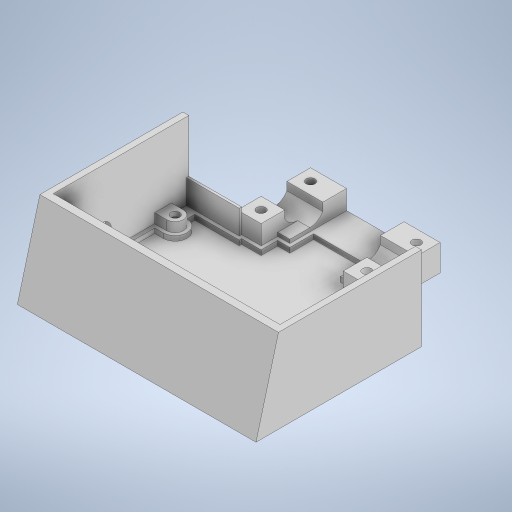
# Autodesk Inventor part: tělo estonsko
Saved by Autodesk Inventor 2024 (Build 280153000, 153)
## iProperties
Created: 2023-09-06
Part Number: tělo estonsko
Material: Všeobecné
Document SubType Name: Modeling
Designer: Simak
Density: 1 g/cm^3
Appearance: Výchozí
Author: Simak
Autodesk Inventor part; units mm, degrees
ref_plane "YZ Plane" through (0, 0, 0) normal (1, 0, 0) x (0, 1, 0)
ref_plane "XZ Plane" through (0, 0, 0) normal (0, 1, 0) x (-1, 0, 0)
ref_plane "XY Plane" through (0, 0, 0) normal (0, 0, 1) x (1, 0, 0)
sketch "Náčrt1" plane through (0, 0, 0) normal (0, 1, 0) x (-1, 0, 0)
  line L0 (49.75, -19.25) -> (49.75, 49.75)
  line L1 (49.75, 49.75) -> (-49.75, 49.75)
  line L2 (-49.75, 49.75) -> (-49.75, -19.25)
  line L3 (-49.75, -19.25) -> (-27, -19.25)
  line L4 (-27, -19.25) -> (-27, -49.75)
  line L5 (-27, -49.75) -> (27, -49.75)
  line L6 (27, -49.75) -> (27, -19.25)
  line L7 (27, -19.25) -> (49.75, -19.25)
  point P0 (0, 0)
  dimension "d0" = 30.5
  dimension "d1" = 99.5
  dimension "d2" = 22.75
  dimension "d3" = 99.5
  dimension "d4" = 54
  dimension "d5" = 49.75
  dimension "d6" = 49.75
  constraints: 16 end point, 6 perpendicular, 2 vertical, 1 parallel
  measures "d0" distance of L3.end L4.end
  measures "d1" distance of L0.end L1.end
  measures "d2" distance of L2.end L3.end
  measures "d3" distance between parallel lines of L1 L5
  measures "d4" distance of L4.end L5.end
  measures "d5" horizontal distance of L1.end point (0, 0)
  measures "d6" distance from line of point (0, 0) L1
extrude "Vysunutí1" add sketch "Náčrt1" along normal blind 3
sketch "Náčrt2" plane through (27, 0, -19.25) normal (1, 0, 0) x (0, 0, -1)
  line L0 (30.5, 3) -> (0, 3)
  line L1 (0, 3) -> (0, 11)
  line L2 (0, 11) -> (9.875, 11)
  line L3 (9.875, 11) -> (9.875, 7.646)
  arc A0 (9.875, 7.646) -> (20.625, 7.646) centre (15.25, 10.582835) ccw
  line L4 (20.625, 7.646) -> (20.625, 11)
  line L5 (20.625, 11) -> (30.5, 11)
  line L6 (30.5, 11) -> (30.5, 3)
  line L7 (0, 0) -> (30.5, 0)
  point P0 (-19.25, 0)
  dimension "d9" = 6.125
  dimension "d10" = 11
  dimension "d11" = 9.875
  dimension "d12" = 3.354
  constraints: 12 end point, 3 perpendicular, 2 equal length, 2 point on circle, 2 point on line, 1 centre point, 1 parallel, 1 vertical
  measures "d9" radius of A0
  measures "d10" distance between parallel lines of L5 L7
  measures "d11" distance of L4.end L5.end
  measures "d12" distance of L4.start L4.end
extrude "Vysunutí2" add sketch "Náčrt2" against normal up to surface (54 mm away)
sketch "Náčrt3" plane through (27, 3, -19.25) normal (0, 0, 1) x (1, 0, 0)
  line L0 (0, 8) -> (-54, 8) projected
  line L1 (-39, 8) -> (-39, 0)
  line L2 (-15, 8) -> (-15, 0)
  line L3 (-76.75, 0) -> (22.75, 0) projected
  line L4 (0, 8) -> (0, 0) projected
  line L5 (-54, 8) -> (-54, 0) projected
  line L6 (-15, 4) -> (0, 4)
  line L7 (-39, 4) -> (-54, 4)
  point P0 (-27, -3)
  dimension "d24" = 24
  constraints: 8 end point, 4 midpoint, 4 point on line, 2 vertical, 1 collinear
  measures "d24" distance between parallel lines of L1 L2
extrude "Vysunutí3" cut sketch "Náčrt3" against normal up to surface (20.625 mm away) contours L2 L3 L1 L0
sketch "Náčrt4" plane through (-27, 3, -19.25) normal (0, 0, 1) x (1, 0, 0)
  line L0 (0, 1.457835) -> (15, 1.457835)
  line L1 (39, 1.457835) -> (54, 1.457835)
  line L2 (9.875, 1.457835) -> (9.875, 8)
  line L3 (54, 8) -> (0, 8)
  line L4 (0, 8) -> (0, 0)
  line L5 (44.125, 8) -> (44.125, 1.457835)
  line L6 (54, 8) -> (54, 0)
  line L7 (15, 0) -> (15, 8)
  line L8 (39, 8) -> (39, 0)
  point P0 (27, -3)
  dimension "d20" = 9.875
  dimension "d21" = 9.875
  constraints: 4 end point, 4 point on line, 2 vertical
  measures "d20" distance between parallel lines of L4 L2
  measures "d21" distance between parallel lines of L6 L5
extrude "Vysunutí4" cut sketch "Náčrt4" against normal up to next contours L2 L3 L7 L0 | L8 L3 L5 L1
sketch "Náčrt5" plane through (-27, 3, -19.25) normal (0, 0, 1) x (1, 0, 0)
  line L0 (9.875, 1.457835) -> (9.875, 0)
  line L1 (15, 0) -> (0, 0)
  line L2 (44.125, 1.457835) -> (44.125, 0)
  line L3 (54, 0) -> (39, 0)
  line L4 (15, 1.457835) -> (9.875, 1.457835)
  line L5 (15, 0) -> (15, 1.457835)
  line L6 (-22.75, 0) -> (76.75, 0)
  line L7 (39, 1.457835) -> (39, 0)
  line L8 (44.125, 1.457835) -> (39, 1.457835)
  point P0 (27, -3)
  constraints: 4 end point, 2 coincident, 2 point on line, 1 parallel, 1 vertical
extrude "Vysunutí5" cut sketch "Náčrt5" against normal blind 6.875
sketch "Náčrt6" plane through (27, 7.646, -39.875) normal (0, 0, 1) x (1, 0, 0)
  line L0 (0, 3.354) -> (-54, 3.354) projected
  line L1 (-37, 3.354) -> (-37, -3.646)
  line L2 (-37, -3.646) -> (-17, -3.646)
  line L3 (-17, -3.646) -> (-17, 3.354)
  line L4 (-76.75, -4.646) -> (22.75, -4.646) projected
  line L5 (0, 3.354) -> (0, 0) projected
  line L6 (-17, -0.146) -> (0, -0.146) construction
  line L7 (-37, -0.146) -> (-54, -0.146) construction
  line L8 (-54, -7.646) -> (-54, 3.354) projected
  point P0 (-27, -7.646)
  dimension "d27" = 1
  dimension "d35" = 20
  constraints: 10 end point, 4 point on line, 2 horizontal, 2 midpoint, 2 perpendicular, 1 collinear, 1 vertical
  measures "d27" distance between parallel lines of L4 L2
  measures "d35" distance of L1.end L2.end
extrude "Vysunutí6" cut sketch "Náčrt6" against normal up to next
sketch "Náčrt7" plane through (-27, 11, -19.25) normal (0, 1, 0) x (1, 0, 0)
  circle A0 centre (4.9375, 4.9375) radius 1.85
  circle A1 centre (4.9375, 25.5625) radius 1.85
  circle A2 centre (49.0625, 25.5625) radius 1.85
  circle A3 centre (49.0625, 4.9375) radius 1.85
  line L0 (76.75, 0) -> (54, 0) projected
  line L1 (49.0625, 4.9375) -> (54, 0) construction
  line L2 (54, 0) -> (44.125, 0) projected
  line L3 (44.125, 0) -> (49.0625, 4.9375) construction
  line L4 (54, 9.875) -> (49.0625, 4.9375) construction
  line L5 (9.875, 0) -> (9.875, 6.875) projected
  line L6 (4.9375, 4.9375) -> (9.875, 0) construction
  line L7 (0, 30.5) -> (0, 0) projected
  line L8 (0, 0) -> (4.9375, 4.9375) construction
  line L9 (4.9375, 4.9375) -> (0, 9.875) construction
  line L10 (0, 20.625) -> (4.9375, 25.5625) construction
  line L11 (4.9375, 25.5625) -> (0, 30.5) construction
  line L12 (54, 0) -> (54, 30.5) projected
  line L13 (54, 20.625) -> (49.0625, 25.5625) construction
  line L14 (49.0625, 25.5625) -> (54, 30.5) construction
  point P0 (27, -19.25)
  dimension "d36" = 3.7
  constraints: 20 end point, 12 equal length, 4 centre point, 3 equal radius, 1 coincident
  measures "d36" diameter of A1
extrude "Vysunutí7" cut sketch "Náčrt7" against normal through all
sketch "Náčrt27" plane through (0, 0, 0) normal (0, -1, 0) x (1, 0, 0)
  circle A0 centre (22.0625, -44.8125) radius 1.85
  line L0 (19.2375, -43.181485) -> (22.0625, -41.550471)
  line L1 (22.0625, -41.550471) -> (24.8875, -43.181485)
  line L2 (24.8875, -43.181485) -> (24.8875, -46.443515)
  line L3 (24.8875, -46.443515) -> (22.0625, -48.074529)
  line L4 (22.0625, -48.074529) -> (19.2375, -46.443515)
  line L5 (19.2375, -46.443515) -> (19.2375, -43.181485)
  line L6 (19.2375, -25.818515) -> (19.2375, -22.556485)
  line L7 (19.2375, -22.556485) -> (22.0625, -20.925471)
  line L8 (22.0625, -20.925471) -> (24.8875, -22.556485)
  line L9 (24.8875, -22.556485) -> (24.8875, -25.818515)
  line L10 (24.8875, -25.818515) -> (22.0625, -27.449529)
  line L11 (22.0625, -27.449529) -> (19.2375, -25.818515)
  circle A1 centre (-22.0625, -24.1875) radius 1.85
  line L12 (-19.2375, -25.818515) -> (-22.0625, -27.449529)
  line L13 (-22.0625, -27.449529) -> (-24.8875, -25.818515)
  line L14 (-24.8875, -25.818515) -> (-24.8875, -22.556485)
  line L15 (-24.8875, -22.556485) -> (-22.0625, -20.925471)
  line L16 (-22.0625, -20.925471) -> (-19.2375, -22.556485)
  line L17 (-19.2375, -22.556485) -> (-19.2375, -25.818515)
  circle A2 centre (-22.0625, -44.8125) radius 1.85
  line L18 (-19.2375, -46.443515) -> (-22.0625, -48.074529)
  line L19 (-22.0625, -48.074529) -> (-24.8875, -46.443515)
  line L20 (-24.8875, -46.443515) -> (-24.8875, -43.181485)
  line L21 (-24.8875, -43.181485) -> (-22.0625, -41.550471)
  line L22 (-22.0625, -41.550471) -> (-19.2375, -43.181485)
  line L23 (-19.2375, -43.181485) -> (-19.2375, -46.443515)
  point P0 (0, 0)
  point P1 (22.0625, -24.1875)
  dimension "d179" = 5.65
  constraints: 48 end point, 4 vertical, 3 coincident, 3 equal length, 1 horizontal alignment, 1 vertical alignment, 52 other
  measures "d179" distance between parallel lines of L2 L5
extrude "Vysunutí30" cut sketch "Náčrt27" against normal blind 7 contours A0 | L0 L1 L2 L3 L4 L5 | L6 L7 L8 L9 L10 L11 | A1 | L12 L13 L14 L15 L16 L17 | A2 | L18 L19 L20 L21 L22 L23
chamfer "Zkosení2" distance 1 angle 45 4 edges at (20.2125, 7, -44.8125) (20.2125, 7, -24.1875) (-23.9125, 7, -24.1875) (-23.9125, 7, -44.8125)
sketch "Náčrt28" plane through (0, 3, 0) normal (0, 1, 0) x (1, 0, 0)
  circle A0 centre (-42.25, 8.5) radius 1.85
  circle A1 centre (42.25, 8.5) radius 1.85
  circle A2 centre (42.25, -29) radius 1.85
  circle A3 centre (-42.25, -29) radius 1.85
  line L0 (-42.25, 8.5) -> (-49.75, 8.5) construction
  line L1 (-49.75, 19.25) -> (-49.75, -49.75) projected
  line L2 (42.25, 8.5) -> (49.75, 8.5) construction
  line L3 (49.75, -49.75) -> (49.75, 19.25) projected
  line L4 (-49.75, -49.75) -> (49.75, -49.75) projected
  point P0 (0, 0)
  dimension "d185" = 3.7
  dimension "d186" = 84.5
  dimension "d187" = 37.5
  dimension "d195" = 20.75
  constraints: 4 centre point, 4 end point, 3 equal radius, 3 point on line, 2 horizontal alignment, 2 vertical alignment, 1 collinear, 1 horizontal
  measures "d185" diameter of A0
  measures "d186" distance of L2.start L0.start
  measures "d187" distance of A3.centre L0.start
  measures "d195" distance from line of L4 A3.centre
sketch "Náčrt29" plane through (49.75, 0, 49.75) normal (1, 0, 0) x (0, 0, -1)
  line L0 (0, 0) -> (69, 0)
  line L1 (0, 0) -> (9.378222, 35)
  line L2 (9.378222, 35) -> (12.48405, 35)
  line L3 (12.48405, 35) -> (3.909676, 3)
  line L4 (0, 3) -> (69, 3)
  line L5 (0, 0) -> (0, 3)
  point P0 (49.75, 0)
  point P1 (0.803848, 3)
  dimension "d188" = 75
  dimension "d189" = 35
  dimension "d190" = 3
  constraints: 6 end point, 1 horizontal, 1 parallel, 1 point on line
  measures "d188" angle of L0 L1
  measures "d189" distance between parallel lines of L0 L2
  measures "d190" distance between parallel lines of L1 L3
extrude "Vysunutí31" add sketch "Náčrt29" against normal up to surface (99.5 mm away) contours L1 L2 L3 L4
extrude "Vysunutí32" cut sketch "Náčrt29" against normal through all contours L5 L4 L1
extrude "Vysunutí33" cut sketch "Náčrt28" against normal up to next
sketch "Náčrt31" plane through (0, 3, 0) normal (0, 1, 0) x (1, 0, 0)
  line L0 (37.136, -36.833) -> (45.136, -36.833)
  line L1 (45.136, -36.833) -> (45.136, -44.833)
  line L2 (45.136, -44.833) -> (37.136, -44.833)
  line L3 (37.136, -44.833) -> (37.136, -36.833)
  line L4 (-4, -36.833) -> (4, -36.833)
  line L5 (4, -36.833) -> (4, -44.833)
  line L6 (4, -44.833) -> (-4, -44.833)
  line L7 (-4, -44.833) -> (-4, -36.833)
  line L8 (-45.463, -36.833) -> (-37.463, -36.833)
  line L9 (-37.463, -36.833) -> (-37.463, -44.833)
  line L10 (-37.463, -44.833) -> (-45.463, -44.833)
  line L11 (-45.463, -44.833) -> (-45.463, -36.833)
  line L12 (49.75, -45.840324) -> (49.75, 19.25)
  line L13 (-49.75, 19.25) -> (-49.75, -45.840324)
  line L14 (-49.75, -49.75) -> (49.75, -49.75)
  point P0 (0, 0)
  point P1 (0, -36.833)
  dimension "d198" = 8
  dimension "d199" = 4.614
  dimension "d200" = 4.287
  dimension "d201" = 4.917
  constraints: 24 end point, 6 parallel, 5 equal length, 3 horizontal, 3 perpendicular, 2 horizontal alignment, 1 midpoint, 1 point on line, 1 vertical alignment
  measures "d198" distance between parallel lines of L2 L0
  measures "d199" distance between parallel lines of L12 L1
  measures "d200" distance between parallel lines of L13 L11
  measures "d201" distance from line of L14 L5.end
extrude "Vysunutí34" cut sketch "Náčrt31" against normal up to next
sketch "Náčrt32" plane through (-27, 0, -19.25) normal (0, 0, -1) x (-1, 0, 0)
  line L0 (0, 0) -> (22.75, 0) projected
  line L1 (22.75, 0) -> (20.25, 0)
  line L2 (20.25, 0) -> (20.25, 35)
  line L3 (20.25, 35) -> (22.75, 35)
  line L4 (22.75, 35) -> (22.75, 0)
  line L5 (-76.75, 0) -> (-74.25, 0)
  line L6 (-74.25, 0) -> (-74.25, 35)
  line L7 (-74.25, 35) -> (-76.75, 35)
  line L8 (-76.75, 35) -> (-76.75, 0)
  line L9 (-76.75, 35) -> (22.75, 35) projected
  point P0 (-27, 0)
  point P1 (20.25, 0)
  dimension "d204" = 2.5
  constraints: 16 end point, 4 parallel, 2 horizontal, 2 perpendicular, 1 collinear, 1 point on line
  measures "d204" distance between parallel lines of L2 L4
extrude "Vysunutí35" add sketch "Náčrt32" against normal up to next
sketch "Náčrt33" plane through (-49.75, 0, -19.25) normal (-1, 0, 0) x (0, 0, 1)
  line L0 (36.318, 10.36) -> (42.098, 10.36) construction
  line L1 (36.318, 8.78) -> (42.098, 8.78)
  line L2 (42.098, 11.94) -> (36.318, 11.94)
  arc A0 (36.318, 11.94) -> (36.318, 8.78) centre (36.318, 10.36) ccw
  arc A1 (42.098, 8.78) -> (42.098, 11.94) centre (42.098, 10.36) ccw
  line L3 (0, 0) -> (69, 0) projected
  line L4 (0, 0) -> (0, 35) projected
  line L5 (36.318, 14.44) -> (42.098, 14.44)
  arc A2 (42.098, 6.28) -> (42.098, 14.44) centre (42.098, 10.36) ccw
  line L6 (42.098, 6.28) -> (36.318, 6.28)
  arc A3 (36.318, 14.44) -> (36.318, 6.28) centre (36.318, 10.36) ccw
  point P0 (19.25, 0)
  point P1 (39.208, 10.36)
  point P2 (34.738, 10.36)
  point P3 (43.678, 10.36)
  dimension "d207" = 8.78
  dimension "d208" = 3.16
  dimension "d209" = 8.94
  dimension "d210" = 34.738
  dimension "d211" = 2.5
  constraints: 12 end point, 10 point on circle, 4 centre point, 4 tangent, 2 parallel, 1 horizontal, 1 midpoint, 3 other
  measures "d207" distance between parallel lines of L3 L1
  measures "d208" distance between parallel lines of L1 L2
  measures "d209" distance of point (34.738, 10.36) point (43.678, 10.36)
  measures "d210" distance from line of L4 point (34.738, 10.36)
  measures "d211" distance between parallel lines of L2 L5
extrude "Vysunutí36" cut sketch "Náčrt33" against normal up to surface (2.5 mm away) contours A0 L2 A1 L1 | L5 A2 L6 A3
sketch "Náčrt34" plane through (0, 3, 0) normal (0, 1, 0) x (1, 0, 0)
  circle A0 centre (42.25, -29) radius 1.85 projected
  circle A1 centre (42.25, 8.5) radius 1.85 projected
  circle A2 centre (-42.25, 8.5) radius 1.85 projected
  circle A3 centre (-42.25, -29) radius 1.85 projected
  circle A4 centre (42.25, -29) radius 3.5
  circle A5 centre (42.25, 8.5) radius 3.5
  circle A6 centre (-42.25, 8.5) radius 3.5
  circle A7 centre (-42.25, -29) radius 3.5
  point P0 (0, 0)
  dimension "d214" = 7
  constraints: 4 centre point, 4 coincident, 3 equal radius
  measures "d214" diameter of A4
extrude "Vysunutí37" add sketch "Náčrt34" along normal blind 4
sketch "Náčrt35" plane through (0, 0, 0) normal (0, -1, 0) x (1, 0, 0)
  line L0 (19.2375, -25.818515) -> (19.2375, -22.556485)
  circle A0 centre (42.25, -8.5) radius 1.85
  line L1 (39.425, -10.131015) -> (39.425, -6.868985)
  line L2 (39.425, -6.868985) -> (42.25, -5.237971)
  line L3 (42.25, -5.237971) -> (45.075, -6.868985)
  line L4 (45.075, -6.868985) -> (45.075, -10.131015)
  line L5 (45.075, -10.131015) -> (42.25, -11.762029)
  line L6 (42.25, -11.762029) -> (39.425, -10.131015)
  circle A1 centre (42.25, 29) radius 1.85
  line L7 (39.425, 27.368985) -> (39.425, 30.631015)
  line L8 (39.425, 30.631015) -> (42.25, 32.262029)
  line L9 (42.25, 32.262029) -> (45.075, 30.631015)
  line L10 (45.075, 30.631015) -> (45.075, 27.368985)
  line L11 (45.075, 27.368985) -> (42.25, 25.737971)
  line L12 (42.25, 25.737971) -> (39.425, 27.368985)
  circle A2 centre (-42.25, 29) radius 1.85
  line L13 (-45.075, 27.368985) -> (-45.075, 30.631015)
  line L14 (-45.075, 30.631015) -> (-42.25, 32.262029)
  line L15 (-42.25, 32.262029) -> (-39.425, 30.631015)
  line L16 (-39.425, 30.631015) -> (-39.425, 27.368985)
  line L17 (-39.425, 27.368985) -> (-42.25, 25.737971)
  line L18 (-42.25, 25.737971) -> (-45.075, 27.368985)
  circle A3 centre (-42.25, -8.5) radius 1.85
  line L19 (-45.075, -10.131015) -> (-45.075, -6.868985)
  line L20 (-45.075, -6.868985) -> (-42.25, -5.237971)
  line L21 (-42.25, -5.237971) -> (-39.425, -6.868985)
  line L22 (-39.425, -6.868985) -> (-39.425, -10.131015)
  line L23 (-39.425, -10.131015) -> (-42.25, -11.762029)
  line L24 (-42.25, -11.762029) -> (-45.075, -10.131015)
  point P0 (0, 0)
  constraints: 48 end point, 4 coincident, 4 equal length, 4 vertical, 52 other
extrude "Vysunutí38" cut sketch "Náčrt35" against normal blind 4 contours A0 | L1 L2 L3 L4 L5 L6 | A1 | L7 L8 L9 L10 L11 L12 | A2 | L13 L14 L15 L16 L17 L18 | A3 | L19 L20 L21 L22 L23 L24
chamfer "Zkosení3" distance 1 angle 45 4 edges at (40.4, 4, -8.5) (40.4, 4, 29) (-44.1, 4, 29) (-44.1, 4, -8.5)
sketch "Náčrt36" plane through (42.25, 7, -8.5) normal (0, 1, 0) x (1, 0, 0)
  circle A0 centre (0, 0) radius 3.5
  line L0 (0, -3.5) -> (5, -3.5)
  line L1 (5, -54.340324) -> (5, 10.75)
  line L2 (0, 3.5) -> (5, 3.5)
  line L3 (0, -34) -> (5, -34)
  circle A1 centre (0, -37.5) radius 3.5
  line L4 (0, -41) -> (5, -41)
  line L5 (-84.5, -41) -> (-89.5, -41)
  line L6 (-89.5, 10.75) -> (-89.5, -54.340324)
  circle A2 centre (-84.5, -37.5) radius 3.5
  line L7 (-84.5, -34) -> (-89.5, -34)
  circle A3 centre (-84.5, 0) radius 3.5
  line L8 (-84.5, -3.5) -> (-89.5, -3.5)
  line L9 (-84.5, 3.5) -> (-89.5, 3.5)
  point P0 (-42.25, -8.5)
  point P1 (-84.5, 3.5)
  point P2 (5, 3.5)
  point P3 (0, 3.5)
  constraints: 16 end point, 8 horizontal, 6 point on line, 4 perpendicular, 4 tangent, 3 parallel, 3 vertical alignment, 2 point on circle, 4 other
extrude "Vysunutí39" add sketch "Náčrt36" against normal up to next contours A0 L2 L1 L0 | L4 A1 L3 L1 | L5 L6 L7 A2 | L9 A3 L8 L6
sketch "Náčrt37" plane through (27, 7.646, -39.875) normal (0, 0, 1) x (1, 0, 0)
  line L0 (-15, -4.646) -> (-39, -4.646)
  line L1 (-15, 0) -> (-15, -4.646)
  line L2 (-39, -4.646) -> (-39, 0)
  line L3 (-39, 0) -> (-39, 3.354)
  line L4 (-37, 3.354) -> (-54, 3.354)
  line L5 (-15, 0) -> (-15, 3.354)
  line L6 (-15, 3.354) -> (-17.006285, 3.354)
  line L7 (-17.006285, 3.354) -> (-37, 3.354)
  point P0 (-27, -7.646)
  constraints: 8 end point, 2 vertical, 1 collinear, 1 perpendicular, 1 point on line
extrude "Vysunutí40" cut sketch "Náčrt37" against normal up to next
sketch "Náčrt40" plane through (47.25, 3, -19.25) normal (-1, 0, 0) x (0, 0, 1)
  line L0 (0, -3) -> (0, 32) projected
  line L1 (0, 0) -> (1, 0)
  line L2 (1, 0) -> (1, 10)
  line L3 (1, 10) -> (0, 10)
  line L4 (0, 10) -> (0, 0)
  line L5 (0, 0) -> (7.25, 0) projected
  point P0 (19.25, -3)
  point P1 (0, 10)
  dimension "d236" = 1
  dimension "d237" = 10
  constraints: 8 end point, 2 parallel, 1 horizontal, 1 perpendicular
  measures "d236" distance of L2.end L3.end
  measures "d237" distance between parallel lines of L5 L3
extrude "Vysunutí41" add sketch "Náčrt40" along normal blind 22
sketch "Náčrt41" plane through (-47.25, 3, -19.25) normal (1, 0, 0) x (0, 0, -1)
  line L0 (-1, 10) -> (0, 10) projected
  line L1 (0, 10) -> (0, 8) projected
  line L2 (0, 0) -> (0, 8) projected
  line L3 (-1, 0) -> (0, 0) projected
  line L4 (-1, 0) -> (-1, 10) projected
  point P0 (-19.25, -3)
extrude "Vysunutí42" add sketch "Náčrt41" along normal blind 22
sketch "Náčrt42" plane through (0, 3, 0) normal (0, 1, 0) x (1, 0, 0)
  line L0 (-25.25, 18.25) -> (-47.25, 18.25)
  line L1 (-47.25, 18.25) -> (-47.25, 12)
  line L2 (-47.25, 12) -> (-42.25, 12)
  arc A0 (-42.25, 5) -> (-42.25, 12) centre (-42.25, 8.5) ccw
  line L3 (-42.25, 5) -> (-47.25, 5)
  line L4 (-47.25, 5) -> (-47.25, -25.5)
  line L5 (-47.25, -25.5) -> (-42.25, -25.5)
  arc A1 (-42.25, -32.5) -> (-42.25, -25.5) centre (-42.25, -29) ccw
  line L6 (-42.25, -32.5) -> (-47.25, -32.5)
  line L7 (-47.25, -32.5) -> (-47.25, -45.840324)
  line L8 (-47.25, -45.840324) -> (47.25, -45.840324)
  line L9 (47.25, -45.840324) -> (47.25, -32.5)
  line L10 (47.25, -32.5) -> (42.25, -32.5)
  arc A2 (42.25, -25.5) -> (42.25, -32.5) centre (42.25, -29) ccw
  line L11 (42.25, -25.5) -> (47.25, -25.5)
  line L12 (47.25, -25.5) -> (47.25, 5)
  line L13 (47.25, 5) -> (42.25, 5)
  arc A3 (42.25, 12) -> (42.25, 5) centre (42.25, 8.5) ccw
  line L14 (42.25, 12) -> (47.25, 12)
  line L15 (47.25, 12) -> (47.25, 18.25)
  line L16 (47.25, 18.25) -> (25.25, 18.25)
  line L17 (25.25, 18.25) -> (25.25, 19.25)
  line L18 (25.25, 19.25) -> (17.125, 19.25)
  line L19 (17.125, 19.25) -> (17.125, 26.125)
  line L20 (17.125, 26.125) -> (12, 26.125)
  line L21 (12, 26.125) -> (12, 49.75)
  line L22 (-12, 49.75) -> (12, 49.75)
  line L23 (-12, 26.125) -> (-12, 49.75)
  line L24 (-12, 26.125) -> (-17.125, 26.125)
  line L25 (-17.125, 19.25) -> (-17.125, 26.125)
  line L26 (-17.125, 19.25) -> (-25.25, 19.25)
  line L27 (-25.25, 19.25) -> (-25.25, 18.25)
  line L28 (-37.463, -36.833) -> (-37.463, -44.833)
  line L29 (-37.463, -44.833) -> (-45.463, -44.833)
  line L30 (-45.463, -44.833) -> (-45.463, -36.833)
  line L31 (-45.463, -36.833) -> (-37.463, -36.833)
  line L32 (4, -36.833) -> (4, -44.833)
  line L33 (4, -44.833) -> (-4, -44.833)
  line L34 (-4, -44.833) -> (-4, -36.833)
  line L35 (-4, -36.833) -> (4, -36.833)
  line L36 (45.136, -36.833) -> (45.136, -44.833)
  line L37 (45.136, -44.833) -> (37.136, -44.833)
  line L38 (37.136, -44.833) -> (37.136, -36.833)
  line L39 (37.136, -36.833) -> (45.136, -36.833)
  line L40 (12, 34.5) -> (17.125, 34.5)
  line L41 (-17.125, 34.5) -> (-12, 34.5)
  line L42 (12, 34.5) -> (-12, 34.5)
  line L43 (45.75, 3.5) -> (45.75, -24)
  line L44 (45.75, -24) -> (42.25, -24)
  arc A4 (42.25, -24) -> (42.25, -34) centre (42.25, -29) ccw
  line L45 (42.25, -34) -> (45.75, -34)
  line L46 (45.75, -34) -> (45.75, -44.340324)
  line L47 (45.75, -44.340324) -> (-45.75, -44.340324)
  line L48 (-45.75, -44.340324) -> (-45.75, -34)
  line L49 (-45.75, -34) -> (-42.25, -34)
  arc A5 (-42.25, -34) -> (-42.25, -24) centre (-42.25, -29) ccw
  line L50 (-42.25, -24) -> (-45.75, -24)
  line L51 (-45.75, -24) -> (-45.75, 3.5)
  line L52 (-45.75, 3.5) -> (-42.25, 3.5)
  arc A6 (-42.25, 3.5) -> (-42.25, 13.5) centre (-42.25, 8.5) ccw
  line L53 (-42.25, 13.5) -> (-45.75, 13.5)
  line L54 (-45.75, 13.5) -> (-45.75, 16.75)
  line L55 (-45.75, 16.75) -> (-23.75, 16.75)
  line L56 (-23.75, 16.75) -> (-23.75, 17.75)
  line L57 (-23.75, 17.75) -> (-15.625, 17.75)
  line L58 (-15.625, 17.75) -> (-15.625, 24.625)
  line L59 (-15.625, 24.625) -> (-10.5, 24.625)
  line L60 (-10.5, 24.625) -> (-10.5, 48.25)
  line L61 (-10.5, 48.25) -> (10.5, 48.25)
  line L62 (10.5, 48.25) -> (10.5, 24.625)
  line L63 (10.5, 24.625) -> (15.625, 24.625)
  line L64 (15.625, 24.625) -> (15.625, 17.75)
  line L65 (15.625, 17.75) -> (23.75, 17.75)
  line L66 (23.75, 17.75) -> (23.75, 16.75)
  line L67 (23.75, 16.75) -> (45.75, 16.75)
  line L68 (45.75, 16.75) -> (45.75, 13.5)
  line L69 (45.75, 13.5) -> (42.25, 13.5)
  arc A7 (42.25, 13.5) -> (42.25, 3.5) centre (42.25, 8.5) ccw
  line L70 (42.25, 3.5) -> (45.75, 3.5)
  line L71 (36.136, -35.833) -> (36.136, -45.833)
  line L72 (36.136, -45.833) -> (46.136, -45.833)
  line L73 (46.136, -45.833) -> (46.136, -35.833)
  line L74 (46.136, -35.833) -> (36.136, -35.833)
  line L75 (5, -35.833) -> (5, -45.833)
  line L76 (5, -45.833) -> (-5, -45.833)
  line L77 (-5, -45.833) -> (-5, -35.833)
  line L78 (-5, -35.833) -> (5, -35.833)
  line L79 (-36.463, -45.833) -> (-36.463, -35.833)
  line L80 (-36.463, -35.833) -> (-46.463, -35.833)
  line L81 (-46.463, -35.833) -> (-46.463, -45.833)
  line L82 (-46.463, -45.833) -> (-36.463, -45.833)
  line L83 (-42.25, -34) -> (-42.25, -35.833)
  line L84 (42.25, -34) -> (42.25, -35.833)
  line L85 (42.25, 13.5) -> (42.25, 16.75)
  line L86 (-42.25, 13.5) -> (-42.25, 16.75)
  point P0 (0, 0)
  point P1 (10.5, 34.5)
  point P2 (-10.5, 34.5)
  point P3 (-36.463, -44.340324)
  point P4 (-5, -44.340324)
  point P5 (5, -44.340324)
  point P6 (36.136, -44.340324)
  dimension "d242" = 1.5
  dimension "d243" = 1
  dimension "d244" = 1
  dimension "d245" = 1
  constraints: 90 end point, 8 point on circle, 6 point on line, 4 centre point, 2 perpendicular, 1 collinear, 40 other
  measures "d242" distance between parallel lines of L12 L43
  measures "d243" distance between parallel lines of L38 L71
  measures "d244" distance between parallel lines of L35 L78
  measures "d245" distance between parallel lines of L28 L79
extrude "Vysunutí43" cut sketch "Náčrt42" against normal blind 2 contours L42 L62 L63 L64 L65 L66 L67 L85 A7 L70 L43 L44 A4 L84 L74 L71 L47 L75 L78 L77 L79 L80 L83 A5 L50 L51 L52 A6 L86 L55 L56 L57 L58 L59 L60
